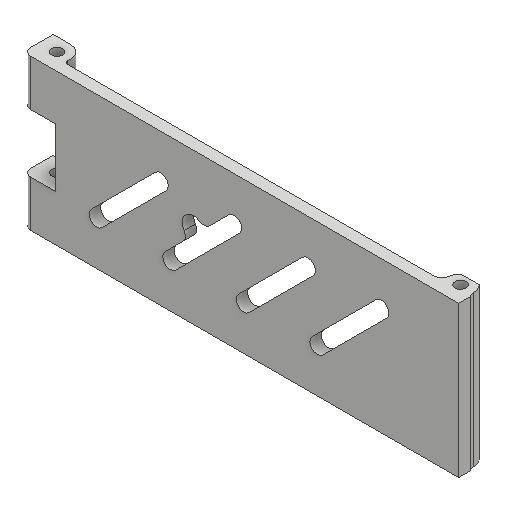
# Autodesk Inventor part: 3DP_PLA_Controller_Case_Side_Wall_Longer
Saved by Autodesk Inventor 2026.1 (Build 301233000, 233)
## iProperties
Created: 2017-05-26
Part Number: 3DP_PLA_Controller_Case_Side_Wall_Longer
Material: Ogólny
Document SubType Name: Modeling
Designer: Andrzej
Density: 1 g/cm^3
Appearance: Domyślna
Author: Andrzej
Autodesk Inventor part; units mm, degrees
ref_plane "YZ Plane" through (0, 0, 0) normal (1, 0, 0) x (0, 1, 0)
ref_plane "XZ Plane" through (0, 0, 0) normal (0, 1, 0) x (-1, 0, 0)
sketch "Szkic1" plane through (0, 0, 0) normal (0, 0, 1) x (1, 0, 0)
  circle A0 centre (-5.5, -12.5) radius 1.5
  circle A1 centre (-5.5, 53.1646) radius 1.5
  circle A2 centre (101.455, -12.5) radius 1.5
  arc A3 (-10, -15) -> (-8, -17) centre (-8, -15) ccw
  line L0 (-8, -17) -> (136.455, -17)
  arc A4 (136.455, -17) -> (141.455, -12) centre (136.455, -12) ccw
  line L1 (141.455, -12) -> (141.455, -2)
  arc A5 (141.455, -2) -> (136.455, 3) centre (136.455, -2) ccw
  line L2 (136.455, 3) -> (127.455, 3)
  arc A6 (115.455, 15) -> (127.455, 3) centre (127.455, 15) ccw
  line L3 (115.455, 15) -> (115.455, 29.1646)
  arc A7 (127.455, 41.1646) -> (115.455, 29.1646) centre (127.455, 29.1646) ccw
  line L4 (127.455, 41.1646) -> (136.455, 41.1646)
  arc A8 (136.455, 41.1646) -> (141.455, 46.1646) centre (136.455, 46.1646) ccw
  line L5 (141.455, 46.1646) -> (141.455, 56.1646)
  arc A9 (141.455, 56.1646) -> (136.455, 61.1646) centre (136.455, 56.1646) ccw
  line L6 (136.455, 61.1646) -> (122.455, 61.1646)
  line L7 (107.455, 76.1646) -> (122.455, 61.1646)
  line L8 (107.455, 76.1646) -> (107.455, 88.1646)
  arc A10 (107.455, 88.1646) -> (102.455, 93.1646) centre (102.455, 88.1646) ccw
  line L9 (102.455, 93.1646) -> (92.455, 93.1646)
  arc A11 (92.455, 93.1646) -> (87.455, 88.1646) centre (92.455, 88.1646) ccw
  line L10 (87.455, 88.1646) -> (87.455, 79.1646)
  arc A12 (75.455, 67.1646) -> (87.455, 79.1646) centre (75.455, 79.1646) ccw
  line L11 (75.455, 67.1646) -> (22, 67.1646)
  arc A13 (10, 79.1646) -> (22, 67.1646) centre (22, 79.1646) ccw
  line L12 (10, 79.1646) -> (10, 88.1646)
  arc A14 (10, 88.1646) -> (5, 93.1646) centre (5, 88.1646) ccw
  line L13 (5, 93.1646) -> (-5, 93.1646)
  arc A15 (-5, 93.1646) -> (-10, 88.1646) centre (-5, 88.1646) ccw
  line L14 (-10, 88.1646) -> (-10, -15)
  circle A16 centre (97.455, 83.1646) radius 2
  circle A17 centre (131.455, -7) radius 2
  circle A18 centre (131.455, 51.1646) radius 2
  circle A19 centre (0, 83.1646) radius 2
  line L15 (89.5711, 35.5361) -> (89.5711, 17.5361)
  arc A20 (83.5711, 11.5361) -> (89.5711, 17.5361) centre (83.5711, 17.5361) ccw
  line L16 (83.5711, 11.5361) -> (78.5711, 11.5361)
  arc A21 (72.5711, 17.5361) -> (78.5711, 11.5361) centre (78.5711, 17.5361) ccw
  line L17 (72.5711, 17.5361) -> (72.5711, 35.5361)
  arc A22 (78.5711, 41.5361) -> (72.5711, 35.5361) centre (78.5711, 35.5361) ccw
  line L18 (78.5711, 41.5361) -> (83.5711, 41.5361)
  arc A23 (89.5711, 35.5361) -> (83.5711, 41.5361) centre (83.5711, 35.5361) ccw
  line L19 (107.455, 22.1646) -> (107.455, 25.6646)
  line L20 (107.455, 25.6646) -> (109.455, 25.6646)
  line L21 (109.455, 25.6646) -> (109.455, 22.1646)
  line L22 (109.455, 22.1646) -> (107.455, 22.1646)
  line L23 (82.5, 60.1646) -> (86, 60.1646)
  line L24 (86, 60.1646) -> (86, 58.1646)
  line L25 (86, 58.1646) -> (82.5, 58.1646)
  line L26 (82.5, 58.1646) -> (82.5, 60.1646)
  line L27 (53.5, 60.1646) -> (57, 60.1646)
  line L28 (57, 60.1646) -> (57, 58.1646)
  line L29 (57, 58.1646) -> (53.5, 58.1646)
  line L30 (53.5, 58.1646) -> (53.5, 60.1646)
  line L31 (24.5, 60.1646) -> (28, 60.1646)
  line L32 (28, 60.1646) -> (28, 58.1646)
  line L33 (28, 58.1646) -> (24.5, 58.1646)
  line L34 (24.5, 58.1646) -> (24.5, 60.1646)
  line L35 (10, 58.1646) -> (10, 60.1646)
  line L36 (10, 60.1646) -> (13.5, 60.1646)
  line L37 (13.5, 60.1646) -> (13.5, 58.1646)
  line L38 (13.5, 58.1646) -> (10, 58.1646)
  line L39 (39, 60.1646) -> (42.5, 60.1646)
  line L40 (42.5, 60.1646) -> (42.5, 58.1646)
  line L41 (42.5, 58.1646) -> (39, 58.1646)
  line L42 (39, 58.1646) -> (39, 60.1646)
  line L43 (68, 60.1646) -> (71.5, 60.1646)
  line L44 (71.5, 60.1646) -> (71.5, 58.1646)
  line L45 (71.5, 58.1646) -> (68, 58.1646)
  line L46 (68, 58.1646) -> (68, 60.1646)
  line L47 (107.455, 37.6646) -> (107.455, 41.1646)
  line L48 (107.455, 41.1646) -> (109.455, 41.1646)
  line L49 (109.455, 41.1646) -> (109.455, 37.6646)
  line L50 (109.455, 37.6646) -> (107.455, 37.6646)
  line L51 (107.455, 6.6646) -> (107.455, 10.1646)
  line L52 (107.455, 10.1646) -> (109.455, 10.1646)
  line L53 (109.455, 10.1646) -> (109.455, 6.6646)
  line L54 (109.455, 6.6646) -> (107.455, 6.6646)
  line L55 (54.7961, 40.5361) -> (54.7961, 12.5361)
  arc A24 (48.7961, 6.5361) -> (54.7961, 12.5361) centre (48.7961, 12.5361) ccw
  line L56 (48.7961, 6.5361) -> (30.7961, 6.5361)
  arc A25 (24.7961, 12.5361) -> (30.7961, 6.5361) centre (30.7961, 12.5361) ccw
  line L57 (24.7961, 12.5361) -> (24.7961, 40.5361)
  arc A26 (30.7961, 46.5361) -> (24.7961, 40.5361) centre (30.7961, 40.5361) ccw
  line L58 (30.7961, 46.5361) -> (48.7961, 46.5361)
  arc A27 (54.7961, 40.5361) -> (48.7961, 46.5361) centre (48.7961, 40.5361) ccw
  circle A28 centre (65.8311, 7.4861) radius 1.6
  circle A29 centre (15.0311, 50.6661) radius 1.6
  circle A30 centre (89.9611, 50.6661) radius 1.6
  circle A31 centre (13.7611, 2.4061) radius 1.6
  circle A32 centre (65.8311, 35.4261) radius 1.6
  circle A33 centre (96.3111, 2.4061) radius 1.6
  line L59 (105.455, -17) -> (105.455, -14)
  line L60 (105.455, -14) -> (-10, -14)
  arc A34 (-2.3377, -14) -> (-8.6623, -14) centre (-5.5, -12.5) ccw
  arc A35 (104.6173, -14) -> (98.2927, -14) centre (101.455, -12.5) ccw
  line L61 (-5.5, -9) -> (-10, -9)
  point P0 (0, 0)
  point P1 (0, 0)
  dimension "d0" = 3
  dimension "d1" = 36
  dimension "d2" = 7
  dimension "d3" = 7
  constraints: 124 end point, 47 point on circle, 36 centre point, 7 point on line, 2 coincident, 2 perpendicular, 1 vertical
  measures "d0" distance between parallel lines of L0 L60
  measures "d1" distance between parallel lines of L1 L59
  measures "d2" diameter of A34
  measures "d3" diameter of A35
extrude "Wyciągnięcie proste1" add sketch "Szkic1" along normal blind 40 contours L60 A34 | L60 L59 L0 A3 L14 | L60 L14 L61 A34 | A35 L60
fillet "Zaokrąglenie1" radius 2 2 edges at (98.2927, -14, 20) (104.6173, -14, 20)
fillet "Zaokrąglenie1" radius 0.8 1 edges at (-2.3377, -14, 20)
sketch "Szkic2" plane through (-8, -17, 0) normal (0, -1, 0) x (1, 0, 0)
  line L0 (0, 0) -> (113.455, 0) projected
  line L1 (113.455, 0) -> (113.455, 40) projected
  line L2 (0, 40) -> (113.455, 40) projected
  line L3 (0, 0) -> (0, 40) projected
  line L4 (-2, 0) -> (-2, 40) projected
  line L5 (-2, 0) -> (-2, 40) projected
  line L6 (-2, 27.75) -> (6.5, 27.75)
  line L7 (6.5, 27.75) -> (6.5, 12.25)
  line L8 (6.5, 12.25) -> (-2, 12.25)
  line L9 (-2, 12.25) -> (-2, 27.75)
  point P0 (8, 0)
  dimension "d7" = 8.5
  dimension "d8" = 15.5
  dimension "d9" = 40
  dimension "d10" = 12.25
  constraints: 8 end point, 2 parallel, 1 horizontal, 1 perpendicular, 1 point on line
  measures "d7" distance of L7.end L8.end
  measures "d8" distance of L6.end L7.end
  measures "d9" distance between parallel lines of L0 L2
  measures "d10" distance between parallel lines of L2 L6
extrude "Wyciągnięcie proste2" cut sketch "Szkic2" against normal through all contours L8 L4 L6 L3 | L3 L6 L7 L8
sketch "Szkic3" plane through (-8, -17, 0) normal (0, -1, 0) x (1, 0, 0)
  line L0 (6.5, 12.25) -> (0, 12.25) projected
  line L1 (0, 0) -> (0, 12.25) projected
  line L2 (0, 0) -> (113.455, 0) projected
  line L3 (113.455, 0) -> (113.455, 40) projected
  line L4 (0, 40) -> (113.455, 40) projected
  line L5 (0, 27.75) -> (0, 40) projected
  line L6 (0, 27.75) -> (6.5, 27.75) projected
  line L7 (6.5, 27.75) -> (6.5, 12.25) projected
  line L8 (103.9778, 0) -> (103.9778, 40) projected
  line L9 (17.5103, 11.5147) -> (34.4808, 28.4853) construction
  line L10 (18.9245, 10.1005) -> (35.8951, 27.0711)
  line L11 (33.0666, 29.8995) -> (16.0961, 12.9289)
  arc A0 (16.0961, 12.9289) -> (18.9245, 10.1005) centre (17.5103, 11.5147) ccw
  arc A1 (35.8951, 27.0711) -> (33.0666, 29.8995) centre (34.4808, 28.4853) ccw
  line L12 (25.9956, 20) -> (49.9956, 20) construction
  line L13 (37.0058, 11.5147) -> (53.9764, 28.4853) construction
  line L14 (38.42, 10.1005) -> (55.3906, 27.0711)
  line L15 (52.5622, 29.8995) -> (35.5916, 12.9289)
  arc A2 (35.5916, 12.9289) -> (38.42, 10.1005) centre (37.0058, 11.5147) ccw
  arc A3 (55.3906, 27.0711) -> (52.5622, 29.8995) centre (53.9764, 28.4853) ccw
  line L16 (45.4911, 20) -> (69.4911, 20) construction
  line L17 (56.5014, 11.5147) -> (73.472, 28.4853) construction
  line L18 (57.9156, 10.1005) -> (74.8862, 27.0711)
  line L19 (72.0577, 29.8995) -> (55.0872, 12.9289)
  arc A4 (55.0872, 12.9289) -> (57.9156, 10.1005) centre (56.5014, 11.5147) ccw
  arc A5 (74.8862, 27.0711) -> (72.0577, 29.8995) centre (73.472, 28.4853) ccw
  line L20 (64.9867, 20) -> (88.9867, 20) construction
  line L21 (75.997, 11.5147) -> (92.9675, 28.4853) construction
  line L22 (77.4112, 10.1005) -> (94.3817, 27.0711)
  line L23 (91.5533, 29.8995) -> (74.5827, 12.9289)
  arc A6 (74.5827, 12.9289) -> (77.4112, 10.1005) centre (75.997, 11.5147) ccw
  arc A7 (94.3817, 27.0711) -> (91.5533, 29.8995) centre (92.9675, 28.4853) ccw
  line L24 (84.4822, 20) -> (108.4822, 20) construction
  arc A8 (45.8917, 23.229) -> (41.926, 19.2633) centre (43.155, 22) ccw
  point P0 (8, 0)
  dimension "d13" = 40
  dimension "d14" = 20
  dimension "d15" = 20
  dimension "d16" = 20
  dimension "d17" = 20
  dimension "d19" = 97.4778
  dimension "d20" = 19.4956
  dimension "d21" = 19.4956
  dimension "d22" = 19.4956
  dimension "d23" = 19.4956
  dimension "d24" = 12
  dimension "d25" = 45
  dimension "d26" = 4
  dimension "d27" = 12
  dimension "d28" = 45
  dimension "d29" = 4
  dimension "d30" = 12
  dimension "d31" = 45
  dimension "d32" = 4
  dimension "d33" = 12
  dimension "d34" = 45
  dimension "d35" = 4
  dimension "d38" = 18
  dimension "d39" = 70.3
  dimension "d40" = 6
  constraints: 40 end point, 18 point on circle, 16 tangent, 9 centre point, 6 parallel, 4 equal length, 4 horizontal, 4 midpoint, 2 point on line, 1 coincident
  measures "d13" distance between parallel lines of L2 L4
  measures "d14" distance from line of L4 L12.start
  measures "d15" distance from line of L4 L16.start
  measures "d16" distance from line of L4 L20.start
  measures "d17" distance from line of L4 L24.start
  measures "d19" distance between parallel lines of L8 L7
  measures "d20" distance from line of L7 L12.start
  measures "d21" distance of L16.start L12.start
  measures "d22" distance of L16.start L20.start
  measures "d23" distance of L20.start L24.start
  measures "d24" distance of L12.start L9.end
  measures "d25" angle of L12 L9
  measures "d26" diameter of A1
  measures "d27" distance of L16.start L13.end
  measures "d28" angle of L16 L13
  measures "d29" diameter of A3
  measures "d30" distance of L20.start L17.end
  measures "d31" angle of L20 L17
  measures "d32" diameter of A5
  measures "d33" distance of L24.start L21.end
  measures "d34" angle of L24 L21
  measures "d35" diameter of A7
  measures "d38" distance from line of L4 point (43.155, 22)
  measures "d39" distance from line of L3 point (43.155, 22)
  measures "d40" diameter of A8
extrude "Wyciągnięcie proste3" cut sketch "Szkic3" against normal through all contours A0 L11 A1 L10 | A2 L15 A3 L14 | A8 L15 | A4 L19 A5 L18 | A6 L23 A7 L22
fillet "Zaokrąglenie2" radius 2 2 edges at (33.926, -15.5, 19.2633) (37.8917, -15.5, 23.229)
ref_plane "Płaszczyzna konstrukcyjna1" through (101.455, -9, 0) normal (0, 1, 0) x (-1, 0, 0)
sketch "Szkic4" plane through (101.455, -9, 0) normal (0, 1, 0) x (-1, 0, 0)
  line L0 (16.8478, 48.5064) -> (-17.7331, 48.5064)
  line L1 (-17.7331, 48.5064) -> (-17.7331, -24.0755)
  line L2 (-17.7331, -24.0755) -> (16.8478, -24.0755)
  line L3 (16.8478, -24.0755) -> (16.8478, 48.5064)
  point P0 (101.455, 0)
  constraints: 8 end point, 2 parallel, 1 horizontal, 1 perpendicular
extrude "Wyciągnięcie proste4" cut sketch "Szkic4" against normal blind 1
equation "\"d10\" = -0.5 * d8 + 0.5 * d9"
equation "\"d16\" = d15"
equation "\"d17\" = d15"
equation "\"d20\" = 0.2 * d19"
equation "\"d21\" = d20"
equation "\"d22\" = d20"
equation "\"d23\" = d20"
